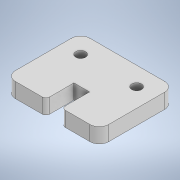
# Autodesk Inventor part: Part147
Saved by Autodesk Inventor 2021.3 (Build 253353000, 353)
## iProperties
Created: 2021-06-26
Part Number: Part147
Material: Generic
Document SubType Name: Modeling
Designer: Fabijan_Sven
Density: 1 g/cm^3
Appearance: Default
Author: Fabijan_Sven
Autodesk Inventor part; units mm, degrees
ref_plane "YZ Plane" through (0, 0, 0) normal (1, 0, 0) x (0, 1, 0)
ref_plane "XZ Plane" through (0, 0, 0) normal (0, 1, 0) x (-1, 0, 0)
ref_plane "XY Plane" through (0, 0, 0) normal (0, 0, 1) x (1, 0, 0)
sketch "Sketch1" plane through (0, 0, 0) normal (0, 1, 0) x (-1, 0, 0)
  line L0 (0, 0) -> (20.2, 0)
  line L1 (50, 0) -> (50, -40)
  line L2 (50, -40) -> (0, -40)
  line L3 (0, -40) -> (0, 0)
  line L4 (20.2, 0) -> (20.2, -15)
  line L5 (20.2, -15) -> (28.6, -15)
  line L6 (28.6, -15) -> (28.6, 0)
  circle A0 centre (40, -30) radius 2.65
  circle A1 centre (10, -30) radius 2.65
  line L7 (28.6, 0) -> (50, 0)
  dimension "d0" = 40
  dimension "d1" = 50
  dimension "d2" = 8.4
  dimension "d3" = 15
  dimension "d4" = 20.2
  dimension "d5" = 5.3
  dimension "d6" = 5.3
  dimension "d7" = 10
  dimension "d8" = 10
  dimension "d9" = 10
  dimension "d10" = 10
  constraints: 16 end point, 4 parallel, 2 centre point, 2 horizontal, 2 perpendicular, 1 point on line
  measures "d0" distance of L1.start L1.end
  measures "d1" distance of L1.end L2.end
  measures "d2" distance of L4.end L5.end
  measures "d3" distance between parallel lines of L0 L5
  measures "d4" distance between parallel lines of L3 L4
  measures "d5" diameter of A0
  measures "d6" diameter of A1
  measures "d7" distance from line of L2 A0.centre
  measures "d8" distance from line of L2 A1.centre
  measures "d9" distance from line of L1 A0.centre
  measures "d10" distance from line of L3 A1.centre
extrude "Extrusion1" add sketch "Sketch1" along normal blind 8
fillet "Fillet1" radius 5 4 edges at (0, 4, -40) (-50, 4, -40) (0, 4, 0) (-50, 4, 0)
fillet "Fillet2" radius 2 2 edges at (-28.6, 4, 0) (-20.2, 4, 0)
body "Solid1"
